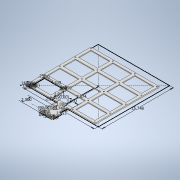
# Autodesk Inventor part: WellPlateFrame - 3L - Part1
Saved by Autodesk Inventor 2020 (Build 240168000, 168)
## iProperties
Created: 2023-02-18
Part Number: WellPlateFrame - 3L - Part1
Material: Generic
Document SubType Name: Modeling
Designer: Beaucage
Density: 1 g/cm^3
Appearance: Default
Author: Beaucage
Autodesk Inventor part; units mm, degrees
ref_plane "YZ Plane" through (0, 0, 0) normal (1, 0, 0) x (0, 1, 0)
ref_plane "XZ Plane" through (0, 0, 0) normal (0, 1, 0) x (-1, 0, 0)
ref_plane "XY Plane" through (0, 0, 0) normal (0, 0, 1) x (1, 0, 0)
sketch "Sketch1" plane through (0, 0, 0) normal (0, 1, 0) x (-1, 0, 0)
  line L0 (0, 0) -> (76.2, 0)
  line L1 (76.2, 0) -> (76.2, -50.8)
  line L2 (76.2, -50.8) -> (0, -50.8)
  line L3 (0, -50.8) -> (0, 0)
  line L4 (38.1, 0) -> (38.1, -6.35)
  line L5 (38.1, -6.35) -> (12.7, -6.35)
  line L6 (38.1, -6.35) -> (63.5, -6.35)
  line L7 (38.1, -6.35) -> (63.5, -6.35) construction
  line L8 (63.5, -6.35) -> (63.5, -19.05)
  line L9 (12.7, -6.35) -> (12.7, -19.05)
  line L10 (63.5, -19.05) -> (63.5, -25.4)
  line L11 (12.7, -19.05) -> (12.7, -25.4)
  line L12 (63.5, -19.05) -> (63.5, -94.05)
  line L13 (63.5, -19.05) -> (138.5, -19.05) construction
  line L14 (12.7, -19.05) -> (12.7, -94.05)
  line L15 (63.5, -94.05) -> (38.1, -94.05)
  line L16 (38.1, -94.05) -> (38.1, -294.05)
  line L17 (38.1, -94.05) -> (238.1, -94.05) construction
  line L18 (238.1, -494.05) -> (-161.9, -494.05)
  line L19 (-161.9, -494.05) -> (-161.9, -94.05)
  line L20 (-161.9, -94.05) -> (238.1, -94.05)
  line L21 (238.1, -94.05) -> (238.1, -494.05)
  line L22 (238.1, -494.05) -> (-161.9, -94.05) construction
  line L23 (-161.9, -494.05) -> (238.1, -94.05) construction
  point P0 (63.5, -50.8)
  point P1 (12.7, -50.8)
  dimension "d0" = 76.2
  dimension "d1" = 50.8
  dimension "d2" = 6.35
  dimension "d3" = 25.4
  dimension "d4" = 25.4
  dimension "d5" = 0
  dimension "d6" = 12.7
  dimension "d7" = 12.7
  dimension "d8" = 6.35
  dimension "d9" = 6.35
  dimension "d10" = 75
  dimension "d11" = 90
  dimension "d12" = 75
  dimension "d13" = 25.4
  dimension "d14" = 200
  dimension "d15" = 90
  dimension "d16" = 400
  dimension "d17" = 400
  constraints: 48 end point, 7 horizontal, 6 vertical, 4 parallel, 4 perpendicular, 3 equal length, 3 midpoint, 1 point on line
  measures "d0" distance of L1.end L2.end
  measures "d1" distance of L0.end L1.end
  measures "d2" distance of L4.start L4.end
  measures "d3" distance of L4.end L5.end
  measures "d4" distance of L4.end L6.end
  measures "d5" distance between parallel lines of L6 L7
  measures "d6" distance of L6.end L8.end
  measures "d7" distance of L5.end L9.end
  measures "d8" distance of L8.end L10.end
  measures "d9" distance of L9.end L11.end
  measures "d10" distance of L8.end L12.end
  measures "d11" angle of L12 L13
  measures "d12" distance of L9.end L14.end
  measures "d13" distance of L12.end L15.end
  measures "d14" distance of L15.end L16.end
  measures "d15" angle of L16 L17
  measures "d16" distance of L19.end L20.end
  measures "d17" distance of L18.end L19.end
extrude "Extrusion1" add sketch "Sketch1" along normal blind 6.35
hole "Hole1" at (-12.7, 0, -6.35) at (-12.7, 0, -19.05) at (-63.5, 0, -6.35) at (-63.5, 0, -19.05) direction (0, 1, 0) diameter 6.604 end through all
sketch "Sketch2" plane through (0, 0, 0) normal (0, -1, 0) x (1, 0, 0)
  line L0 (-238.1, -94.05) -> (-63.5, -94.05) projected
  line L1 (-238.1, -94.05) -> (-238.1, -100.4)
  line L2 (-238.1, -94.05) -> (-231.75, -94.05) construction
  line L3 (-238.1, -100.4) -> (-231.75, -100.4)
  line L4 (-231.75, -100.4) -> (-225.4, -100.4)
  line L5 (-225.4, -100.4) -> (-225.4, -106.75)
  line L6 (-225.4, -106.75) -> (-115.2, -106.75)
  line L7 (-115.2, -106.75) -> (-115.2, -180.75)
  line L8 (-115.2, -180.75) -> (-225.4, -180.75)
  line L9 (-225.4, -180.75) -> (-225.4, -106.75)
  line L10 (-115.2, -106.75) -> (-115.2, -100.4)
  line L11 (-115.2, -100.4) -> (-108.85, -100.4)
  line L12 (-225.4, -180.75) -> (-231.75, -180.75)
  line L13 (-231.75, -180.75) -> (-231.75, -187.1)
  line L14 (-115.2, -180.75) -> (-115.2, -187.1)
  line L15 (-115.2, -187.1) -> (-108.85, -187.1)
  line L16 (-225.4, -106.75) -> (-225.4, -114.75)
  line L17 (-225.4, -106.75) -> (-217.4, -106.75) construction
  line L18 (-225.4, -106.75) -> (-223.4, -106.75)
  line L19 (-223.4, -106.75) -> (-223.4, -108.75)
  line L20 (-223.4, -108.75) -> (-225.4, -108.75)
  line L21 (-225.4, -108.75) -> (-225.4, -106.75)
  line L22 (-115.2, -180.75) -> (-117.2, -180.75)
  line L23 (-117.2, -180.75) -> (-117.2, -178.75)
  line L24 (-117.2, -178.75) -> (-115.2, -178.75)
  line L25 (-115.2, -178.75) -> (-115.2, -180.75)
  line L26 (-223.4, -108.75) -> (-117.2, -108.75)
  line L27 (-117.2, -108.75) -> (-117.2, -178.75)
  line L28 (-117.2, -178.75) -> (-223.4, -178.75)
  line L29 (-223.4, -178.75) -> (-223.4, -108.75)
  point P0 (0, 0)
  dimension "d27" = 6.35
  dimension "d28" = 90
  dimension "d29" = 6.35
  dimension "d30" = 6.35
  dimension "d31" = 6.35
  dimension "d32" = 110.2
  dimension "d33" = 74
  dimension "d34" = 6.35
  dimension "d35" = 6.35
  dimension "d36" = 6.35
  dimension "d37" = 6.35
  dimension "d38" = 6.35
  dimension "d39" = 8
  dimension "d40" = 90
  dimension "d41" = 2
  dimension "d42" = 2
  dimension "d43" = 2
  dimension "d44" = 2
  constraints: 58 end point, 11 perpendicular, 8 horizontal, 8 parallel, 4 vertical
  measures "d27" distance of L0.start L1.end
  measures "d28" angle of L1 L2
  measures "d29" distance of L1.end L3.end
  measures "d30" distance of L3.end L4.end
  measures "d31" distance of L4.end L5.end
  measures "d32" distance of L7.end L8.end
  measures "d33" distance of L6.end L7.end
  measures "d34" distance of L10.end L11.end
  measures "d35" distance of L8.end L12.end
  measures "d36" distance of L12.end L13.end
  measures "d37" distance of L7.end L14.end
  measures "d38" distance of L14.end L15.end
  measures "d39" distance of L5.end L16.end
  measures "d40" angle of L16 L17
  measures "d41" distance of L19.end L20.end
  measures "d42" distance of L18.end L19.end
  measures "d43" distance of L23.end L24.end
  measures "d44" distance of L22.end L23.end
extrude "Extrusion2" cut sketch "Sketch2" against normal through all contours L26 L27 L28 L29
hole "Hole2" at (-231.75, 0, -100.4) at (-231.75, 0, -187.1) at (-108.85, 0, -100.4) at (-108.85, 0, -187.1) direction (0, 1, 0) diameter 5.1562 end through all
extrude "Extrusion3" cut sketch "Sketch2" against normal blind 2 contours L6 L19 L20 L9 | L6 L7 L24 L27 L26 L19 | L20 L29 L28 L23 L8 L9 | L7 L8 L23 L24
pattern_linear "Rectangular Pattern1" count 3 spacing 122.9106 along (1, 0, 0) count 4 spacing 86.9442 along (0, 0, -1) of "Extrusion2", "Hole2", "Extrusion3"
sketch "Sketch3" plane through (0, 0, 0) normal (0, -1, 0) x (1, 0, 0)
  circle A0 centre (136.9712, -447.9326) radius 2.5781 projected
  line L0 (136.9712, -447.9326) -> (143.3212, -447.9326)
  line L1 (143.3212, -447.9326) -> (143.3212, -454.2826)
  line L2 (143.3212, -454.2826) -> (136.9712, -454.2826)
  line L3 (136.9712, -454.2826) -> (136.9712, -447.9326)
  line L4 (-12.7, -94.05) -> (161.9, -94.05) projected
  line L5 (143.3212, -454.2826) -> (161.9, -454.2826)
  line L6 (161.9, -454.2826) -> (161.9, -94.05)
  line L7 (161.9, -94.05) -> (143.3212, -94.05)
  line L8 (143.3212, -94.05) -> (143.3212, -454.2826)
  line L9 (161.9, -454.2826) -> (-238.1, -454.2826)
  line L10 (-238.1, -454.2826) -> (-238.1, -500.3541)
  line L11 (-238.1, -500.3541) -> (161.9, -500.3541)
  line L12 (161.9, -500.3541) -> (161.9, -454.2826)
  point P0 (0, 0)
  dimension "d62" = 6.35
  dimension "d63" = 6.35
  constraints: 24 end point, 6 parallel, 3 horizontal, 3 perpendicular
  measures "d62" distance of L1.end L2.end
  measures "d63" distance of L0.end L1.end
extrude "Extrusion4" cut sketch "Sketch3" against normal through all contours L8 L4 L6 L5 L1 | L2 L5 L12 L11 L10 L9
body "Solid1"
